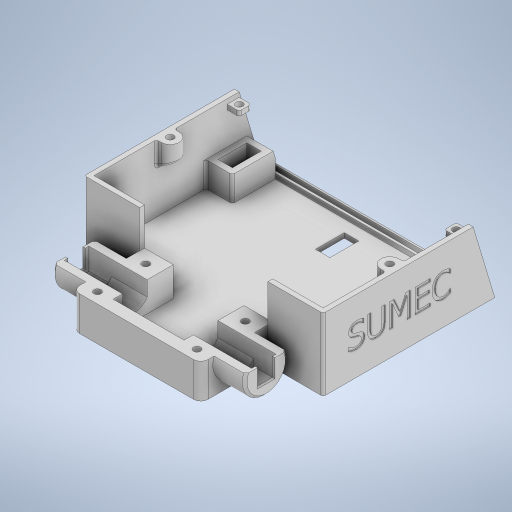
# Autodesk Inventor part: Tělo POKUS
Saved by Autodesk Inventor 2024 (Build 280153000, 153)
## iProperties
Created: 2023-04-15
Part Number: Tělo POKUS
Material: Všeobecné
Document SubType Name: Modeling
Designer: 42060
Density: 1 g/cm^3
Appearance: Výchozí
Author: 42060
Autodesk Inventor part; units mm, degrees
ref_plane "YZ Plane" through (0, 0, 0) normal (1, 0, 0) x (0, 1, 0)
ref_plane "XZ Plane" through (0, 0, 0) normal (0, 1, 0) x (-1, 0, 0)
ref_plane "XY Plane" through (0, 0, 0) normal (0, 0, 1) x (1, 0, 0)
sketch "Základ" plane through (0, 0, 0) normal (0, 0, 1) x (1, 0, 0)
  line L0 (0, 0) -> (49.75, 0)
  line L1 (49.75, 0) -> (49.75, -71.5)
  line L2 (49.75, -71.5) -> (26.75, -71.5)
  line L3 (26.75, -99.5) -> (0, -99.5)
  line L4 (0, -99.5) -> (0, 0)
  line L5 (0, -10) -> (47.75, -10)
  line L6 (47.75, -10) -> (47.75, -69.5)
  line L7 (47.75, -69.5) -> (14.75, -69.5)
  line L8 (14.75, -69.5) -> (14.75, -94.5)
  line L9 (14.75, -94.5) -> (0, -94.5)
  line L10 (26.75, -71.5) -> (26.75, -80.375)
  line L11 (26.75, -80.375) -> (26.75, -90.625)
  line L12 (26.75, -90.625) -> (26.75, -99.5)
  line L13 (26.75, -90.625) -> (14.75, -90.625)
  line L14 (26.75, -80.375) -> (14.75, -80.375)
  line L15 (26.75, -71.5) -> (26.75, -69.5)
  dimension "d0" = 49.75
  dimension "d1" = 99.5
  dimension "d3" = 2
  dimension "d5" = 28
  dimension "d14" = 10.25
  dimension "d15" = 12
  dimension "d16" = 5
  dimension "d17" = 23
  dimension "d18" = 2
  dimension "d19" = 10
  constraints: 32 end point, 8 perpendicular, 6 point on line, 3 horizontal, 2 collinear, 1 parallel, 1 vertical
  measures "d0" distance of L0.start L0.end
  measures "d1" distance between parallel lines of L3 L0
  measures "d3" distance between parallel lines of L1 L6
  measures "d5" distance of L2.end L3.start
  measures "d14" distance of L10.end L11.end
  measures "d15" distance between parallel lines of L8 L10
  measures "d16" distance between parallel lines of L9 L3
  measures "d17" distance between parallel lines of L1 L12
  measures "d18" distance between parallel lines of L2 L7
  measures "d19" distance between parallel lines of L0 L5
extrude "Podlaha" add sketch "Základ" along normal blind 2 contours L5 L6 L7 L8 L9 L4
extrude "Stěny" add sketch "Základ" along normal blind 30 contours L0 L1 L2 L15 L7 L6 L5 L4
extrude "Zadní stěny" add sketch "Základ" along normal blind 15 contours L9 L8 L13 L12 L3 L4 | L10 L14 L8 L7 L15
extrude "Stěna pod motorem" add sketch "Základ" along normal blind 5.25 contours L11 L13 L8 L14
sketch "Náčrt2" plane through (49.75, -71.5, 0) normal (1, 0, 0) x (0, 0, -1)
  line L0 (-2, 61.5) -> (-30, 61.5) projected
  line L1 (-2, 61.5) -> (-30, 61.5) projected
  line L2 (-30, 0) -> (-30, 71.5) projected
  line L3 (0, 71.5) -> (-30, 71.5) projected
  line L4 (0, 71.5) -> (0, 0) projected
  line L5 (-30, 62.5) -> (-10, 68.5)
  line L6 (-10, 68.5) -> (0, 71.5)
  dimension "d28" = 1
  dimension "d30" = 20
  constraints: 4 end point, 1 collinear, 1 point on line
  measures "d28" distance from line of L5.start L0
  measures "d30" horizontal distance of L5.end L5.start
extrude "Rampa" cut sketch "Náčrt2" against normal through all
sketch "Náčrt3" plane through (0, -10, 2) normal (-1, 0, 0) x (0, 0, 1)
  line L0 (0, 0) -> (28, 0) projected
  line L1 (0, 0) -> (28, 0) projected
  line L2 (24.3731, 0) -> (7.5, 5.0619)
  line L3 (7.5, 5.0619) -> (0, 5.0619)
  line L4 (0, 5.0619) -> (0, 0)
  line L5 (28, 1) -> (-2, 10) projected
  point P0 (-2, 10)
  point P1 (2, 7)
  point P2 (24.3731, 0)
  dimension "d34" = 7.5
  dimension "d37" = 2
  constraints: 6 end point, 1 horizontal, 1 perpendicular, 1 point on line, 2 other
  measures "d34" distance of L2.end L3.end
extrude "Přední rampa" cut sketch "Náčrt3" against normal up to surface (47.75 mm away)
sketch "Držák motoru" plane through (14.75, -94.5, 2) normal (-1, 0, 0) x (0, 0, 1)
  line L0 (3.25, 14.125) -> (13, 14.125) projected
  line L1 (3.25, 14.125) -> (3.25, 3.875) projected
  line L2 (3.25, 3.875) -> (13, 3.875) projected
  line L3 (6.13, 14.125) -> (12.37, 14.125)
  line L4 (12.37, 3.875) -> (6.13, 3.875)
  line L5 (3.25, 3.875) -> (13, 3.875) projected
  arc A0 (12.37, 3.875) -> (12.37, 14.125) centre (9.25, 9) ccw
  arc A1 (6.13, 14.125) -> (6.13, 3.875) centre (9.25, 9) ccw
  line L6 (15.25, 14.125) -> (15.25, 3.875) construction
  circle A2 centre (9.25, 9) radius 9
  line L7 (9.25, 18) -> (0, 18)
  line L8 (0, 0) -> (0, 89.5619) projected
  line L9 (0, 0) -> (13, 0) projected
  line L10 (13, -5) -> (13, 3.875) projected
  line L11 (0, 0) -> (13, 0) projected
  line L12 (0, 0) -> (13, 0) projected
  line L13 (12.37, 14.125) -> (12.37, 17.4419)
  line L14 (12.37, 3.875) -> (12.37, 0.5581)
  line L15 (12.37, 0.5581) -> (12.37, 0)
  line L16 (12.37, 17.4419) -> (12.37, 18)
  line L17 (12.37, 18) -> (9.25, 18)
  point P0 (-2, 94.5)
  point P1 (15.25, 9)
  point P2 (15.25, 9)
  point P3 (3.25, 9)
  point P4 (3.25, 9)
  point P5 (6.13, 3.875)
  point P6 (9.25, 0)
  point P7 (16.7333, 14)
  point P8 (16.7333, 4)
  point P9 (12.37, 0)
  dimension "d38" = 6
  dimension "d39" = 6
  dimension "d41" = 3
  dimension "d48" = 12
  constraints: 18 end point, 9 point on circle, 7 point on line, 4 tangent, 3 centre point, 3 coincident, 3 vertical, 2 horizontal alignment, 2 midpoint, 1 horizontal, 1 perpendicular
  measures "d38" radius of A0
  measures "d39" radius of A1
  measures "d41" radial gap between concentric circles of A2 A0
  measures "d48" distance between parallel lines of L1 L6
sketch "Náčrt10" plane through (14.75, -99.5, 0) normal (1, 0, 0) x (0, 0, -1)
  line L0 (-5.25, 8.875) -> (-15, 8.875) construction
  line L1 (-5.25, 8.875) -> (-17.25, 8.875) construction
  line L2 (-17.25, 8.875) -> (-17.25, 19.125) construction
  line L3 (-17.25, 19.125) -> (-5.25, 19.125) construction
  line L4 (-5.25, 19.125) -> (-5.25, 8.875) construction
  line L5 (-14.37, 8.875) -> (-8.13, 8.875)
  arc A0 (-8.13, 8.875) -> (-8.13, 19.125) centre (-11.25, 14) ccw
  line L6 (-14.37, 19.125) -> (-8.13, 19.125)
  arc A1 (-14.37, 5.5581) -> (-14.37, 22.4419) centre (-11.25, 14) ccw
  line L7 (-14.37, 8.875) -> (-14.37, 5.5581)
  line L8 (-14.37, 19.125) -> (-14.37, 22.4419)
  point P0 (0, 99.5)
  point P1 (-11.25, 19.125)
  point P2 (-11.25, 19.125)
  point P3 (-11.25, 8.875)
  point P4 (-11.25, 8.875)
  dimension "d79" = 12
  dimension "d80" = 6
  dimension "d81" = 18
  constraints: 16 end point, 5 point on line, 4 midpoint, 4 point on circle, 3 coincident, 2 centre point, 2 parallel, 2 perpendicular, 2 vertical alignment, 1 collinear, 1 horizontal, 1 horizontal alignment, 1 tangent
  measures "d79" distance between parallel lines of L4 L2
  measures "d80" radius of A0
  measures "d81" diameter of A1
extrude "Držák motoru (kulaté)" add sketch "Náčrt10" along normal blind 15
sketch "Náčrt11" plane through (29.75, -99.5, 0) normal (1, 0, 0) x (0, 0, -1)
  arc A0 (-8.13, 8.875) -> (-8.13, 19.125) centre (-11.25, 14) ccw projected
  circle A1 centre (-11.25, 14) radius 9
  line L0 (-17.25, 8.875) -> (-5.25, 8.875)
  line L1 (-5.25, 8.875) -> (-5.25, 19.125)
  line L2 (-5.25, 19.125) -> (-17.25, 19.125)
  line L3 (-17.25, 19.125) -> (-17.25, 8.875)
  line L4 (-17.25, 8.875) -> (-5.25, 19.125) construction
  line L5 (-5.25, 8.875) -> (-17.25, 19.125) construction
  line L6 (-14.37, 8.875) -> (-14.37, 5.5581) projected
  line L7 (-14.37, 22.4419) -> (-14.37, 19.125) projected
  point P0 (0, 99.5)
  dimension "d84" = 18
  constraints: 12 end point, 2 midpoint, 2 parallel, 1 centre point, 1 coincident, 1 horizontal, 1 horizontal alignment, 1 perpendicular, 1 tangent
  measures "d84" diameter of A1
extrude "Držák motoru (hranaté)" add sketch "Náčrt11" along normal blind 9.25 contours L0 L1 L2 L7 A1 L6
sketch "Spodní senzory" plane through (0, 0, 2) normal (0, 0, 1) x (1, 0, 0)
  line L0 (0, -4.9381) -> (47.75, -4.9381) projected
  line L1 (0, -94.5) -> (0, -4.9381) projected
  line L2 (0, -94.5) -> (14.75, -94.5) projected
  line L3 (14.75, -94.5) -> (14.75, -69.5) projected
  line L4 (14.75, -69.5) -> (47.75, -69.5) projected
  line L5 (47.75, -69.5) -> (47.75, -4.9381) projected
  line L6 (0, -24.4381) -> (5.5, -24.4381)
  line L7 (0, -21.9381) -> (3, -21.9381)
  line L8 (3, -21.9381) -> (3, -9.9381)
  line L9 (3, -9.9381) -> (0, -9.9381)
  line L10 (0, -7.4381) -> (5.5, -7.4381)
  line L11 (5.5, -7.4381) -> (5.5, -24.4381)
  line L12 (47.75, -22.8381) -> (36.75, -22.8381)
  line L13 (36.75, -22.8381) -> (36.75, -4.9381)
  line L14 (45.25, -20.3381) -> (39.25, -20.3381)
  line L15 (39.25, -20.3381) -> (39.25, -8.3381)
  line L16 (39.25, -8.3381) -> (45.25, -8.3381)
  line L17 (45.25, -8.3381) -> (45.25, -20.3381)
  point P0 (0, 0)
  dimension "d155" = 3
  dimension "d157" = 12
  dimension "d159" = 2.5
  dimension "d163" = 5
  dimension "d170" = 2.5
  dimension "d171" = 2.5
  dimension "d174" = 2.5
  dimension "d175" = 2.5
  dimension "d176" = 2.5
  dimension "d177" = 12
  dimension "d178" = 6
  dimension "d179" = 3.4
  constraints: 24 end point, 6 point on line, 5 perpendicular, 4 horizontal, 2 parallel, 1 vertical
  measures "d155" distance of L7.start L7.end
  measures "d157" distance of L7.end L8.end
  measures "d159" distance between parallel lines of L7 L6
  measures "d163" distance between parallel lines of L0 L9
  measures "d170" distance between parallel lines of L10 L9
  measures "d171" distance between parallel lines of L8 L11
  measures "d174" distance between parallel lines of L13 L15
  measures "d175" distance between parallel lines of L5 L17
  measures "d176" distance between parallel lines of L14 L12
  measures "d177" distance of L14.end L15.end
  measures "d178" distance of L14.start L14.end
  measures "d179" distance between parallel lines of L0 L16
extrude "Spodní senzory (díra)" cut sketch "Spodní senzory" against normal through all contours L9 L8 L7 L1 | L14 L15 L16 L17
extrude "Spodní senzory zvýšení" add sketch "Spodní senzory" along normal blind 10.5 contours L0 L5 L12 L13
sketch "Náčrt12" plane through (0, 0, 15) normal (0, 0, 1) x (1, 0, 0)
  line L0 (26.75, -80.375) -> (26.75, -71.5) projected
  line L1 (26.75, -69.5) -> (26.75, -71.5) projected
  line L2 (26.75, -69.5) -> (14.75, -69.5) projected
  line L3 (14.75, -69.5) -> (14.75, -80.375) projected
  line L4 (14.75, -80.375) -> (26.75, -80.375) projected
  line L5 (26.75, -99.5) -> (26.75, -90.625) projected
  line L6 (26.75, -90.625) -> (14.75, -90.625) projected
  line L7 (14.75, -90.625) -> (14.75, -94.5) projected
  line L8 (14.75, -94.5) -> (0, -94.5) projected
  line L9 (0, -94.5) -> (0, -99.5) projected
  line L10 (0, -99.5) -> (26.75, -99.5) projected
  point P0 (0, 0)
extrude "Vyrovnání držáku motoru" cut sketch "Náčrt12" against normal up to surface (0.63 mm away)
sketch "Náčrt13" plane through (14.75, -80.375, 14.37) normal (0, 0, 1) x (1, 0, 0)
  line L0 (0, 0) -> (0, 10.875) projected
  line L1 (0, 10.875) -> (12, 10.875) projected
  line L2 (0, -14.125) -> (0, -10.25) projected
  line L3 (0, -10.25) -> (24.25, -10.25) projected
  point P0 (-14.75, 80.375)
  point P1 (6, 5.4375)
  point P2 (6, -14.6875)
  dimension "d89" = 6
  dimension "d90" = 5.4375
  dimension "d91" = 6
  dimension "d92" = 4.4375
  measures "d89" distance from line of L0 point (6, 5.438)
  measures "d90" distance from line of L1 point (6, 5.438)
  measures "d91" distance from line of L2 point (6, -14.687)
  measures "d92" distance from line of L3 point (6, -14.687)
hole "Díry pro objímku motoru" at (20.75, -95.0625, 14.37) at (20.75, -74.9375, 14.37) direction (0, 0, -1) diameter 3 depth 6
fillet "Zaoblení stěny motoru" radius 3 1 edges at (26.75, -99.5, 7.185)
fillet "Zaoblení stěny" radius 1 1 edges at (49.75, -71.5, 15)
sketch "Náčrt14" plane through (39, -99.5, 0) normal (1, 0, 0) x (0, 0, -1)
  line L0 (-14.37, 19.125) -> (-5.25, 19.125) projected
  line L1 (-5.25, 19.125) -> (-5.25, 8.875) projected
  line L2 (-5.25, 8.875) -> (-14.37, 8.875) projected
  line L3 (-14.37, 8.875) -> (-14.37, 5.5581) projected
  arc A0 (-14.37, 5.5581) -> (-14.37, 22.4419) centre (-11.25, 14) ccw projected
  line L4 (-14.37, 22.4419) -> (-14.37, 19.125) projected
  line L5 (-14.37, 10.375) -> (-6.75, 10.375)
  line L6 (-6.75, 10.375) -> (-6.75, 17.625)
  line L7 (-6.75, 17.625) -> (-14.37, 17.625)
  line L8 (-14.37, 8.875) -> (-14.37, 10.375)
  line L9 (-14.37, 17.625) -> (-14.37, 19.125)
  point P0 (0, 99.5)
  dimension "d108" = 1.5
  dimension "d109" = 1.5
  dimension "d110" = 1.5
  constraints: 10 end point, 2 perpendicular, 2 point on line, 2 vertical, 2 vertical alignment
  measures "d108" distance between parallel lines of L5 L2
  measures "d109" distance between parallel lines of L1 L6
  measures "d110" distance between parallel lines of L0 L7
extrude "Vysunutí koncovky motoru" add sketch "Náčrt14" along normal blind 1
chamfer "Zkosení držáku motoru" distance 1 angle 45 1 edges at (40, -85.5, 2.25)
chamfer "Toleranční zkosení motoru" distance 0.25 angle 45 2 edges at (29.75, -88.4394, 6.0193) (29.75, -82.5606, 6.0193)
sketch "Náčrt16" plane through (0, 0, 30) normal (0, 0, 1) x (1, 0, 0)
  line L0 (47.75, -36) -> (45.75, -36)
  arc A0 (45.75, -36) -> (45.75, -43.5) centre (45.75, -39.75) ccw
  line L1 (45.75, -43.5) -> (47.75, -43.5)
  line L2 (47.75, -10) -> (47.75, -69.5) projected
  point P0 (47.75, -39.75)
  point P1 (47.75, -39.75)
  point P2 (47.75, -39.75)
  dimension "d130" = 3.75
  dimension "d131" = 2
  constraints: 4 end point, 3 midpoint, 2 coincident, 2 point on circle, 2 point on line, 2 tangent, 1 centre point, 1 horizontal, 1 horizontal alignment, 1 parallel
  measures "d130" radius of A0
  measures "d131" distance of L1.start L1.end
extrude "Vysunutí držáku PCB" add sketch "Náčrt16" against normal blind 10
sketch "Náčrt17" plane through (0, 0, 30) normal (0, 0, 1) x (1, 0, 0)
  arc A0 (45.75, -36) -> (45.75, -43.5) centre (45.75, -39.75) ccw projected
  point P0 (0, 0)
  constraints: 1 coincident
hole "Díra držáku PCB" at (45.75, -39.75, 30) direction (0, 0, -1) diameter 3 depth 6
sketch "Náčrt18" plane through (45.75, -43.5, 30) normal (0, -1, 0) x (1, 0, 0)
  line L0 (-10.625, -22) -> (-25.625, -22) projected
  line L1 (-3.75, -10) -> (0, -10) projected
  line L2 (0, -10) -> (2, -10) projected
  line L3 (-3.75, 0) -> (-3.75, -10) projected
  line L4 (-3.75, -6.6802) -> (2, -10)
  point P0 (-45.75, -30)
  dimension "d141" = 30
  constraints: 2 end point, 1 point on line
  measures "d141" angle of L1 L4
extrude "Zkosení PCB držáku" cut sketch "Náčrt18" against normal blind 10
fillet "Zaoblení hran" radius 1 9 edges at (46.75, -43.5, 20.5774) (46.75, -36, 20.5774) (43.0983, -42.4017, 22.6856) (43.0983, -37.0983, 22.6856) (47.75, -43.5, 25) (47.75, -36, 25) (47.75, -39.75, 20) (36.75, -22.8381, 7.25) (47.75, -22.8381, 7.25)
sketch "Náčrt23" plane through (0, -10, 30) normal (-1, 0, 0) x (0, 0, 1)
  line L0 (-30, 0.0619) -> (-28, 0.0619) projected
  line L1 (-28, 0.0619) -> (-28, 5.0619) projected
  line L2 (-28, 5.0619) -> (-20.5, 5.0619) projected
  line L3 (-20.5, 5.0619) -> (-3.6269, 0) projected
  line L4 (-3.6269, 0) -> (0, 0) projected
  line L5 (0, 1) -> (0, 0) projected
  line L6 (0, 1) -> (-30, 10) projected
  line L7 (-30, 10) -> (-30, 0.0619) projected
  line L8 (-28, 5.0619) -> (-20.5, 5.0619) projected
  line L9 (-26, 5.0619) -> (-26, 6.0619)
  line L10 (-26, 6.0619) -> (-28, 6.0619)
  line L11 (-28, 6.0619) -> (-28, 8.0619)
  line L12 (-28, 8.0619) -> (-26, 8.0619)
  line L13 (-26, 8.0619) -> (-26, 8.8)
  dimension "d187" = 2
  dimension "d188" = 1
  dimension "d189" = 2
  constraints: 10 end point, 4 perpendicular, 4 point on line, 1 vertical alignment
  measures "d187" distance between parallel lines of L1 L9
  measures "d188" distance between parallel lines of L2 L10
  measures "d189" distance between parallel lines of L10 L12
extrude "Vysunutí25" cut sketch "Náčrt23" against normal up to surface (47.75 mm away) contours L6 L5 L4 L3 L2 L9 L10 L11 L12 L13
ref_plane "Pracovní rovina2" through (0, 0, 28) normal (0, 0, 1) x (1, 0, 0)
sketch "Náčrt24" plane through (0, 0, 28) normal (0, 0, 1) x (1, 0, 0)
  line L0 (49.75, -9) -> (47.75, -9) projected
  line L1 (47.75, -9) -> (42.75, -9)
  line L2 (42.75, -9) -> (42.75, -14)
  line L3 (42.75, -14) -> (47.75, -14)
  line L4 (47.75, -14) -> (47.75, -9)
  point P0 (0, 0)
  dimension "d193" = 5
  dimension "d194" = 5
  constraints: 8 end point, 2 parallel, 1 horizontal, 1 perpendicular
  measures "d193" distance of L2.end L3.end
  measures "d194" distance of L1.end L2.end
extrude "Vysunutí26" add sketch "Náčrt24" against normal blind 2
sketch "Náčrt25" plane through (0, 0, 28) normal (0, 0, 1) x (1, 0, 0)
  line L0 (42.75, -9) -> (42.75, -14) projected
  line L1 (42.75, -14) -> (47.75, -14) projected
  point P0 (0, 0)
  point P1 (45.25, -11.5)
  dimension "d197" = 2.5
  dimension "d198" = 2.5
  measures "d197" distance from line of L0 point (45.25, -11.5)
  measures "d198" distance from line of L1 point (45.25, -11.5)
hole "Díra3" at (45.25, -11.5, 28) direction (0, 0, -1) diameter 3 depth 6
fillet "Zaoblení4" radius 1 2 edges at (42.75, -14, 27) (42.75, -9, 27)
mirror "Zrcadlení těla" about plane through (0, 0, 0) normal (1, 0, 0)
sketch "Náčrt15" plane through (49.75, -70.5, 0) normal (1, 0, 0) x (0, 0, -1)
  line L0 (-20.5, 9) -> (-20.5, 54) construction
  line L1 (-20.5, 54) -> (-9.5, 54) construction
  line L2 (-9.5, 54) -> (-9.5, 9) construction
  line L3 (-9.5, 9) -> (-20.5, 9) construction
  line L4 (-30, -1) -> (0, -1) projected
  line L5 (0, 0) -> (0, 70.5) projected
  spline S0 degree 2 poles (-10.1434, 12.8006) (-10.1434, 11.7147) (-10.5972, 10.1912) (-10.9214, 9.5186) knots 0 0 0 1 2 2 2
  line L6 (-10.9214, 9.5186) -> (-12.5908, 9.5186)
  line L7 (-12.5908, 9.5186) -> (-12.5908, 9.6159)
  spline S1 degree 2 poles (-12.5908, 9.6159) (-11.9749, 10.2723) (-11.2942, 11.9335) (-11.2942, 12.7034) knots 0 0 0 1 2 2 2
  spline S2 degree 2 poles (-11.2942, 12.7034) (-11.2942, 13.8055) (-12.2099, 14.9319) (-12.9635, 14.9319) knots 0 0 0 1 2 2 2
  spline S3 degree 2 poles (-12.9635, 14.9319) (-13.5632, 14.9319) (-14.3088, 14.3404) (-14.4951, 13.7002) knots 0 0 0 1 2 2 2
  spline S4 degree 2 poles (-14.4951, 13.7002) (-14.6248, 13.2382) (-14.8031, 12.4684) (-14.9489, 11.893) knots 0 0 0 1 2 2 2
  spline S5 degree 2 poles (-14.9489, 11.893) (-15.0867, 11.3744) (-15.5, 10.5559) (-15.8323, 10.2399) knots 0 0 0 1 2 2 2
  spline S6 degree 2 poles (-15.8323, 10.2399) (-16.1645, 9.9319) (-17.0559, 9.5916) (-17.6394, 9.5916) knots 0 0 0 1 2 2 2
  spline S7 degree 2 poles (-17.6394, 9.5916) (-18.8549, 9.5916) (-20.5, 11.4878) (-20.5, 12.9546) knots 0 0 0 1 2 2 2
  spline S8 degree 2 poles (-20.5, 12.9546) (-20.5, 13.7974) (-20.1677, 15.2885) (-19.8517, 15.9287) knots 0 0 0 1 2 2 2
  line L8 (-19.8517, 15.9287) -> (-18.2634, 15.9287)
  line L9 (-18.2634, 15.9287) -> (-18.2634, 15.8314)
  spline S9 degree 2 poles (-18.2634, 15.8314) (-18.701, 15.3533) (-19.3493, 13.8622) (-19.3493, 13.0438) knots 0 0 0 1 2 2 2
  spline S10 degree 2 poles (-19.3493, 13.0438) (-19.3493, 12.1199) (-18.4822, 10.9773) (-17.7771, 10.9773) knots 0 0 0 1 2 2 2
  spline S11 degree 2 poles (-17.7771, 10.9773) (-17.1451, 10.9773) (-16.3914, 11.6499) (-16.2212, 12.282) knots 0 0 0 1 2 2 2
  spline S12 degree 2 poles (-16.2212, 12.282) (-16.1078, 12.7034) (-15.816, 13.9271) (-15.6945, 14.3323) knots 0 0 0 1 2 2 2
  spline S13 degree 2 poles (-15.6945, 14.3323) (-15.3784, 15.3614) (-14.1062, 16.3177) (-13.1742, 16.3177) knots 0 0 0 1 2 2 2
  spline S14 degree 2 poles (-13.1742, 16.3177) (-12.5827, 16.3177) (-11.4481, 15.8395) (-11.0511, 15.41) knots 0 0 0 1 2 2 2
  spline S15 degree 2 poles (-11.0511, 15.41) (-10.6135, 14.9319) (-10.1434, 13.7164) (-10.1434, 12.8006) knots 0 0 0 1 2 2 2
  spline S16 degree 2 poles (-10.111, 21.1637) (-10.111, 20.2804) (-10.5729, 18.9676) (-11.0348, 18.5057) knots 0 0 0 1 2 2 2
  spline S17 degree 2 poles (-11.0348, 18.5057) (-11.5535, 17.9789) (-13.0122, 17.5494) (-14.0818, 17.5494) knots 0 0 0 1 2 2 2
  line L10 (-14.0818, 17.5494) -> (-20.3217, 17.5494)
  line L11 (-20.3217, 17.5494) -> (-20.3217, 18.8784)
  line L12 (-20.3217, 18.8784) -> (-14.0818, 18.8784)
  spline S18 degree 2 poles (-14.0818, 18.8784) (-13.3849, 18.8784) (-12.4449, 19.0567) (-12.064, 19.3079) knots 0 0 0 1 2 2 2
  spline S19 degree 2 poles (-12.064, 19.3079) (-11.6588, 19.5754) (-11.2455, 20.4992) (-11.2455, 21.1637) knots 0 0 0 1 2 2 2
  spline S20 degree 2 poles (-11.2455, 21.1637) (-11.2455, 21.7877) (-11.6588, 22.7601) (-12.064, 23.0276) knots 0 0 0 1 2 2 2
  spline S21 degree 2 poles (-12.064, 23.0276) (-12.4449, 23.2788) (-13.3768, 23.4571) (-14.0494, 23.4571) knots 0 0 0 1 2 2 2
  line L13 (-14.0494, 23.4571) -> (-20.3217, 23.4571)
  line L14 (-20.3217, 23.4571) -> (-20.3217, 24.7861)
  line L15 (-20.3217, 24.7861) -> (-14.0818, 24.7861)
  spline S22 degree 2 poles (-14.0818, 24.7861) (-13.0365, 24.7861) (-11.5454, 24.3647) (-11.0348, 23.8298) knots 0 0 0 1 2 2 2
  spline S23 degree 2 poles (-11.0348, 23.8298) (-10.5648, 23.3517) (-10.111, 22.0875) (-10.111, 21.1637) knots 0 0 0 1 2 2 2
  line L16 (-10.3217, 35.2642) -> (-10.3217, 33.9352)
  line L17 (-10.3217, 33.9352) -> (-18.936, 33.9352)
  line L18 (-18.936, 33.9352) -> (-13.077, 31.3258)
  line L19 (-13.077, 31.3258) -> (-13.077, 30.5154)
  line L20 (-13.077, 30.5154) -> (-18.936, 27.9303)
  line L21 (-18.936, 27.9303) -> (-10.3217, 27.9303)
  line L22 (-10.3217, 27.9303) -> (-10.3217, 26.6904)
  line L23 (-10.3217, 26.6904) -> (-20.3217, 26.6904)
  line L24 (-20.3217, 26.6904) -> (-20.3217, 28.5057)
  line L25 (-20.3217, 28.5057) -> (-14.7545, 31.0016)
  line L26 (-14.7545, 31.0016) -> (-20.3217, 33.4165)
  line L27 (-20.3217, 33.4165) -> (-20.3217, 35.2642)
  line L28 (-20.3217, 35.2642) -> (-10.3217, 35.2642)
  line L29 (-10.3217, 37.2901) -> (-20.3217, 37.2901)
  line L30 (-20.3217, 37.2901) -> (-20.3217, 43.5462)
  line L31 (-20.3217, 43.5462) -> (-19.1386, 43.5462)
  line L32 (-19.1386, 43.5462) -> (-19.1386, 38.6191)
  line L33 (-19.1386, 38.6191) -> (-16.3995, 38.6191)
  line L34 (-16.3995, 38.6191) -> (-16.3995, 43.2139)
  line L35 (-16.3995, 43.2139) -> (-15.2164, 43.2139)
  line L36 (-15.2164, 43.2139) -> (-15.2164, 38.6191)
  line L37 (-15.2164, 38.6191) -> (-11.5049, 38.6191)
  line L38 (-11.5049, 38.6191) -> (-11.5049, 43.5462)
  line L39 (-11.5049, 43.5462) -> (-10.3217, 43.5462)
  line L40 (-10.3217, 43.5462) -> (-10.3217, 37.2901)
  spline S24 degree 2 poles (-10.1434, 48.9109) (-10.1434, 47.9384) (-10.7998, 46.2934) (-11.4562, 45.6937) knots 0 0 0 1 2 2 2
  spline S25 degree 2 poles (-11.4562, 45.6937) (-12.1045, 45.094) (-14.0494, 44.4376) (-15.3136, 44.4376) knots 0 0 0 1 2 2 2
  spline S26 degree 2 poles (-15.3136, 44.4376) (-16.5697, 44.4376) (-18.4335, 45.0778) (-19.1224, 45.6856) knots 0 0 0 1 2 2 2
  spline S27 degree 2 poles (-19.1224, 45.6856) (-19.795, 46.2853) (-20.5, 47.9222) (-20.5, 48.9352) knots 0 0 0 1 2 2 2
  spline S28 degree 2 poles (-20.5, 48.9352) (-20.5, 49.4376) (-20.3541, 50.3209) (-20.2407, 50.6937) knots 0 0 0 1 2 2 2
  spline S29 degree 2 poles (-20.2407, 50.6937) (-20.1353, 51.0178) (-19.8355, 51.6904) (-19.6572, 52.0227) knots 0 0 0 1 2 2 2
  line L41 (-19.6572, 52.0227) -> (-18.0527, 52.0227)
  line L42 (-18.0527, 52.0227) -> (-18.0527, 51.9173)
  spline S30 degree 2 poles (-18.0527, 51.9173) (-18.2147, 51.7391) (-18.6686, 51.188) (-18.8874, 50.7909) knots 0 0 0 1 2 2 2
  spline S31 degree 2 poles (-18.8874, 50.7909) (-19.0981, 50.41) (-19.3655, 49.5105) (-19.3655, 48.9271) knots 0 0 0 1 2 2 2
  spline S32 degree 2 poles (-19.3655, 48.9271) (-19.3655, 48.2869) (-18.8387, 47.1442) (-18.3363, 46.7147) knots 0 0 0 1 2 2 2
  spline S33 degree 2 poles (-18.3363, 46.7147) (-17.8258, 46.2934) (-16.278, 45.8233) (-15.3136, 45.8233) knots 0 0 0 1 2 2 2
  spline S34 degree 2 poles (-15.3136, 45.8233) (-14.2844, 45.8233) (-12.8015, 46.3177) (-12.2909, 46.7472) knots 0 0 0 1 2 2 2
  spline S35 degree 2 poles (-12.2909, 46.7472) (-11.7966, 47.1686) (-11.2942, 48.295) (-11.2942, 48.9271) knots 0 0 0 1 2 2 2
  spline S36 degree 2 poles (-11.2942, 48.9271) (-11.2942, 49.5024) (-11.5778, 50.483) (-11.7885, 50.8639) knots 0 0 0 1 2 2 2
  spline S37 degree 2 poles (-11.7885, 50.8639) (-11.9992, 51.2285) (-12.4368, 51.7715) (-12.5908, 51.9254) knots 0 0 0 1 2 2 2
  line L43 (-12.5908, 51.9254) -> (-12.5908, 52.0227)
  line L44 (-12.5908, 52.0227) -> (-11.0024, 52.0227)
  spline S38 degree 2 poles (-11.0024, 52.0227) (-10.8485, 51.6904) (-10.5648, 51.107) (-10.4352, 50.6937) knots 0 0 0 1 2 2 2
  spline S39 degree 2 poles (-10.4352, 50.6937) (-10.2893, 50.2561) (-10.1434, 49.5105) (-10.1434, 48.9109) knots 0 0 0 1 2 2 2
  point P0 (-15, 9)
  point P1 (-15, -1)
  point P2 (-9.5, 31.5)
  point P3 (0, 35.25)
  dimension "d145" = 11
  dimension "d146" = 45
  dimension "d185" = 10
  constraints: 4 midpoint, 1 vertical alignment, 2 other
  measures "d145" distance of L0.end L1.end
  measures "d146" distance of L1.end L2.end
  measures "d185" distance between parallel lines of L4 L3
emboss "Nápis SUMEC" sketch "Náčrt15" operation cut depth 0.4 direction (-1, 0, 0)
sketch "Náčrt19" plane through (-49.75, -70.5, 0) normal (-1, 0, 0) x (0, 0, 1)
  line L0 (20.5, 54) -> (20.5, 9) construction
  line L1 (20.5, 9) -> (9.5, 9) construction
  line L2 (9.5, 9) -> (9.5, 54) construction
  line L3 (9.5, 54) -> (20.5, 54) construction
  line L4 (30, -1) -> (0, -1) projected
  line L5 (0, 0) -> (0, 70.5) projected
  spline S0 degree 2 poles (10.1434, 50.1994) (10.1434, 51.2853) (10.5972, 52.8088) (10.9214, 53.4814) knots 0 0 0 1 2 2 2
  line L6 (10.9214, 53.4814) -> (12.5908, 53.4814)
  line L7 (12.5908, 53.4814) -> (12.5908, 53.3841)
  spline S1 degree 2 poles (12.5908, 53.3841) (11.9749, 52.7277) (11.2942, 51.0665) (11.2942, 50.2966) knots 0 0 0 1 2 2 2
  spline S2 degree 2 poles (11.2942, 50.2966) (11.2942, 49.1945) (12.2099, 48.0681) (12.9635, 48.0681) knots 0 0 0 1 2 2 2
  spline S3 degree 2 poles (12.9635, 48.0681) (13.5632, 48.0681) (14.3088, 48.6596) (14.4951, 49.2998) knots 0 0 0 1 2 2 2
  spline S4 degree 2 poles (14.4951, 49.2998) (14.6248, 49.7618) (14.8031, 50.5316) (14.9489, 51.107) knots 0 0 0 1 2 2 2
  spline S5 degree 2 poles (14.9489, 51.107) (15.0867, 51.6256) (15.5, 52.4441) (15.8323, 52.7601) knots 0 0 0 1 2 2 2
  spline S6 degree 2 poles (15.8323, 52.7601) (16.1645, 53.0681) (17.0559, 53.4084) (17.6394, 53.4084) knots 0 0 0 1 2 2 2
  spline S7 degree 2 poles (17.6394, 53.4084) (18.8549, 53.4084) (20.5, 51.5122) (20.5, 50.0454) knots 0 0 0 1 2 2 2
  spline S8 degree 2 poles (20.5, 50.0454) (20.5, 49.2026) (20.1677, 47.7115) (19.8517, 47.0713) knots 0 0 0 1 2 2 2
  line L8 (19.8517, 47.0713) -> (18.2634, 47.0713)
  line L9 (18.2634, 47.0713) -> (18.2634, 47.1686)
  spline S9 degree 2 poles (18.2634, 47.1686) (18.701, 47.6467) (19.3493, 49.1378) (19.3493, 49.9562) knots 0 0 0 1 2 2 2
  spline S10 degree 2 poles (19.3493, 49.9562) (19.3493, 50.8801) (18.4822, 52.0227) (17.7771, 52.0227) knots 0 0 0 1 2 2 2
  spline S11 degree 2 poles (17.7771, 52.0227) (17.1451, 52.0227) (16.3914, 51.3501) (16.2212, 50.718) knots 0 0 0 1 2 2 2
  spline S12 degree 2 poles (16.2212, 50.718) (16.1078, 50.2966) (15.816, 49.0729) (15.6945, 48.6677) knots 0 0 0 1 2 2 2
  spline S13 degree 2 poles (15.6945, 48.6677) (15.3784, 47.6386) (14.1062, 46.6823) (13.1742, 46.6823) knots 0 0 0 1 2 2 2
  spline S14 degree 2 poles (13.1742, 46.6823) (12.5827, 46.6823) (11.4481, 47.1605) (11.0511, 47.59) knots 0 0 0 1 2 2 2
  spline S15 degree 2 poles (11.0511, 47.59) (10.6135, 48.0681) (10.1434, 49.2836) (10.1434, 50.1994) knots 0 0 0 1 2 2 2
  spline S16 degree 2 poles (10.111, 41.8363) (10.111, 42.7196) (10.5729, 44.0324) (11.0348, 44.4943) knots 0 0 0 1 2 2 2
  spline S17 degree 2 poles (11.0348, 44.4943) (11.5535, 45.0211) (13.0122, 45.4506) (14.0818, 45.4506) knots 0 0 0 1 2 2 2
  line L10 (14.0818, 45.4506) -> (20.3217, 45.4506)
  line L11 (20.3217, 45.4506) -> (20.3217, 44.1216)
  line L12 (20.3217, 44.1216) -> (14.0818, 44.1216)
  spline S18 degree 2 poles (14.0818, 44.1216) (13.3849, 44.1216) (12.4449, 43.9433) (12.064, 43.6921) knots 0 0 0 1 2 2 2
  spline S19 degree 2 poles (12.064, 43.6921) (11.6588, 43.4246) (11.2455, 42.5008) (11.2455, 41.8363) knots 0 0 0 1 2 2 2
  spline S20 degree 2 poles (11.2455, 41.8363) (11.2455, 41.2123) (11.6588, 40.2399) (12.064, 39.9724) knots 0 0 0 1 2 2 2
  spline S21 degree 2 poles (12.064, 39.9724) (12.4449, 39.7212) (13.3768, 39.5429) (14.0494, 39.5429) knots 0 0 0 1 2 2 2
  line L13 (14.0494, 39.5429) -> (20.3217, 39.5429)
  line L14 (20.3217, 39.5429) -> (20.3217, 38.2139)
  line L15 (20.3217, 38.2139) -> (14.0818, 38.2139)
  spline S22 degree 2 poles (14.0818, 38.2139) (13.0365, 38.2139) (11.5454, 38.6353) (11.0348, 39.1702) knots 0 0 0 1 2 2 2
  spline S23 degree 2 poles (11.0348, 39.1702) (10.5648, 39.6483) (10.111, 40.9125) (10.111, 41.8363) knots 0 0 0 1 2 2 2
  line L16 (10.3217, 27.7358) -> (10.3217, 29.0648)
  line L17 (10.3217, 29.0648) -> (18.936, 29.0648)
  line L18 (18.936, 29.0648) -> (13.077, 31.6742)
  line L19 (13.077, 31.6742) -> (13.077, 32.4846)
  line L20 (13.077, 32.4846) -> (18.936, 35.0697)
  line L21 (18.936, 35.0697) -> (10.3217, 35.0697)
  line L22 (10.3217, 35.0697) -> (10.3217, 36.3096)
  line L23 (10.3217, 36.3096) -> (20.3217, 36.3096)
  line L24 (20.3217, 36.3096) -> (20.3217, 34.4943)
  line L25 (20.3217, 34.4943) -> (14.7545, 31.9984)
  line L26 (14.7545, 31.9984) -> (20.3217, 29.5835)
  line L27 (20.3217, 29.5835) -> (20.3217, 27.7358)
  line L28 (20.3217, 27.7358) -> (10.3217, 27.7358)
  line L29 (10.3217, 25.7099) -> (20.3217, 25.7099)
  line L30 (20.3217, 25.7099) -> (20.3217, 19.4538)
  line L31 (20.3217, 19.4538) -> (19.1386, 19.4538)
  line L32 (19.1386, 19.4538) -> (19.1386, 24.3809)
  line L33 (19.1386, 24.3809) -> (16.3995, 24.3809)
  line L34 (16.3995, 24.3809) -> (16.3995, 19.7861)
  line L35 (16.3995, 19.7861) -> (15.2164, 19.7861)
  line L36 (15.2164, 19.7861) -> (15.2164, 24.3809)
  line L37 (15.2164, 24.3809) -> (11.5049, 24.3809)
  line L38 (11.5049, 24.3809) -> (11.5049, 19.4538)
  line L39 (11.5049, 19.4538) -> (10.3217, 19.4538)
  line L40 (10.3217, 19.4538) -> (10.3217, 25.7099)
  spline S24 degree 2 poles (10.1434, 14.0891) (10.1434, 15.0616) (10.7998, 16.7066) (11.4562, 17.3063) knots 0 0 0 1 2 2 2
  spline S25 degree 2 poles (11.4562, 17.3063) (12.1045, 17.906) (14.0494, 18.5624) (15.3136, 18.5624) knots 0 0 0 1 2 2 2
  spline S26 degree 2 poles (15.3136, 18.5624) (16.5697, 18.5624) (18.4335, 17.9222) (19.1224, 17.3144) knots 0 0 0 1 2 2 2
  spline S27 degree 2 poles (19.1224, 17.3144) (19.795, 16.7147) (20.5, 15.0778) (20.5, 14.0648) knots 0 0 0 1 2 2 2
  spline S28 degree 2 poles (20.5, 14.0648) (20.5, 13.5624) (20.3541, 12.6791) (20.2407, 12.3063) knots 0 0 0 1 2 2 2
  spline S29 degree 2 poles (20.2407, 12.3063) (20.1353, 11.9822) (19.8355, 11.3096) (19.6572, 10.9773) knots 0 0 0 1 2 2 2
  line L41 (19.6572, 10.9773) -> (18.0527, 10.9773)
  line L42 (18.0527, 10.9773) -> (18.0527, 11.0827)
  spline S30 degree 2 poles (18.0527, 11.0827) (18.2147, 11.2609) (18.6686, 11.812) (18.8874, 12.2091) knots 0 0 0 1 2 2 2
  spline S31 degree 2 poles (18.8874, 12.2091) (19.0981, 12.59) (19.3655, 13.4895) (19.3655, 14.0729) knots 0 0 0 1 2 2 2
  spline S32 degree 2 poles (19.3655, 14.0729) (19.3655, 14.7131) (18.8387, 15.8558) (18.3363, 16.2853) knots 0 0 0 1 2 2 2
  spline S33 degree 2 poles (18.3363, 16.2853) (17.8258, 16.7066) (16.278, 17.1767) (15.3136, 17.1767) knots 0 0 0 1 2 2 2
  spline S34 degree 2 poles (15.3136, 17.1767) (14.2844, 17.1767) (12.8015, 16.6823) (12.2909, 16.2528) knots 0 0 0 1 2 2 2
  spline S35 degree 2 poles (12.2909, 16.2528) (11.7966, 15.8314) (11.2942, 14.705) (11.2942, 14.0729) knots 0 0 0 1 2 2 2
  spline S36 degree 2 poles (11.2942, 14.0729) (11.2942, 13.4976) (11.5778, 12.517) (11.7885, 12.1361) knots 0 0 0 1 2 2 2
  spline S37 degree 2 poles (11.7885, 12.1361) (11.9992, 11.7715) (12.4368, 11.2285) (12.5908, 11.0746) knots 0 0 0 1 2 2 2
  line L43 (12.5908, 11.0746) -> (12.5908, 10.9773)
  line L44 (12.5908, 10.9773) -> (11.0024, 10.9773)
  spline S38 degree 2 poles (11.0024, 10.9773) (10.8485, 11.3096) (10.5648, 11.893) (10.4352, 12.3063) knots 0 0 0 1 2 2 2
  spline S39 degree 2 poles (10.4352, 12.3063) (10.2893, 12.7439) (10.1434, 13.4895) (10.1434, 14.0891) knots 0 0 0 1 2 2 2
  point P0 (15, 9)
  point P1 (15, -1)
  point P2 (9.5, 31.5)
  point P3 (0, 35.25)
  dimension "d149" = 11
  dimension "d150" = 45
  dimension "d186" = 10
  constraints: 4 midpoint, 1 vertical alignment, 2 other
  measures "d149" distance of L0.end L1.end
  measures "d150" distance of L1.end L2.end
  measures "d186" distance between parallel lines of L4 L1
emboss "Nápis SUMEC 2" sketch "Náčrt19" operation cut depth 0.4 direction (1, 0, 0)
